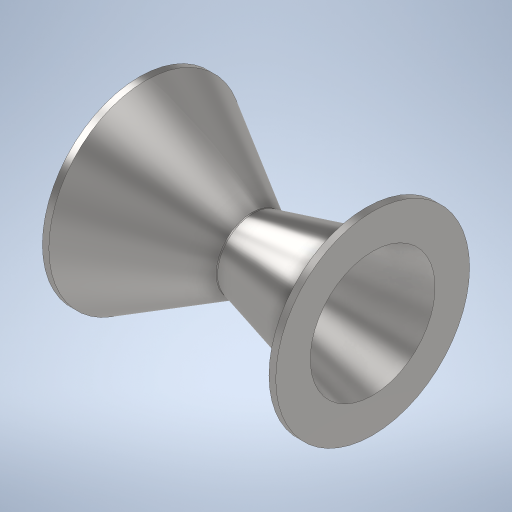
# Autodesk Inventor part: stainless steel final nozzle
Saved by Autodesk Inventor 2023 (Build 270158000, 158)
## iProperties
Created: 2022-09-19
Part Number: stainless steel final nozzle
Material: Stainless Steel
Document SubType Name: Modeling
Designer: station
Density: 8 g/cm^3
Appearance: Semi-Polished
Author: station
Autodesk Inventor part; units mm, degrees
ref_plane "YZ Plane" through (0, 0, 0) normal (1, 0, 0) x (0, 1, 0)
ref_plane "XZ Plane" through (0, 0, 0) normal (0, 1, 0) x (-1, 0, 0)
ref_plane "XY Plane" through (0, 0, 0) normal (0, 0, 1) x (1, 0, 0)
sketch "Sketch1" plane through (0, 0, 0) normal (0, 0, 1) x (1, 0, 0)
  line L0 (0, 0) -> (0, 54.375) construction
  line L1 (0, 54.375) -> (192, 54.375) construction
  line L2 (254.7886, 18.124) -> (254.7886, 0) construction
  line L3 (192, 54.375) -> (254.7886, 18.124)
  line L4 (0, 0) -> (487.78, 0)
  line L5 (254.7886, 18.124) -> (256.7886, 18.124)
  line L6 (256.7886, 18.124) -> (327.1228, 36.97)
  line L7 (327.1228, 36.97) -> (327.1228, 0)
  line L8 (327.1228, 40.0758) -> (256.3936, 21.124)
  line L9 (256.3936, 21.124) -> (255.5924, 21.124)
  line L10 (255.5924, 21.124) -> (192.8038, 57.375)
  line L11 (189, 57.375) -> (189, 54.375)
  line L12 (192, 54.375) -> (189, 54.375)
  line L13 (192, 57.375) -> (189, 57.375)
  line L14 (192, 57.375) -> (192.8038, 57.375)
  line L15 (327.1228, 36.97) -> (327.1228, 40.0758)
  line L16 (327.1228, 57.375) -> (327.1228, 40.0758)
  line L17 (327.1228, 57.375) -> (323.1228, 57.375)
  line L18 (323.1228, 57.375) -> (323.1228, 39.004)
  dimension "d0" = 54.375
  dimension "d1" = 192
  dimension "d2" = 18.124
  dimension "d4" = 30
  dimension "d5" = 18.124
  dimension "d6" = 2
  dimension "d7" = 15
  dimension "d8" = 36.97
  dimension "d9" = 3
  dimension "d10" = 3
  dimension "d14" = 4
  constraints: 38 end point, 4 point on line, 3 horizontal, 2 perpendicular, 2 vertical, 1 parallel
  measures "d0" distance of L0.start L0.end
  measures "d1" distance of L0.end L1.end
  measures "d2" distance of L2.start L2.end
  measures "d4" angle of L4 L3
  measures "d5" distance from line of L4 L2.start
  measures "d6" distance of L2.start L5.end
  measures "d7" angle of L4 L6
  measures "d8" distance of L6.end L7.end
  measures "d9" distance between parallel lines of L3 L10
  measures "d10" distance between parallel lines of L12 L13
  measures "d14" distance of L16.start L17.end
revolve "Revolution1" add sketch "Sketch1" angle 360 about axis through (0, 0, 0) along (1, 0, 0)
body "Solid1"
